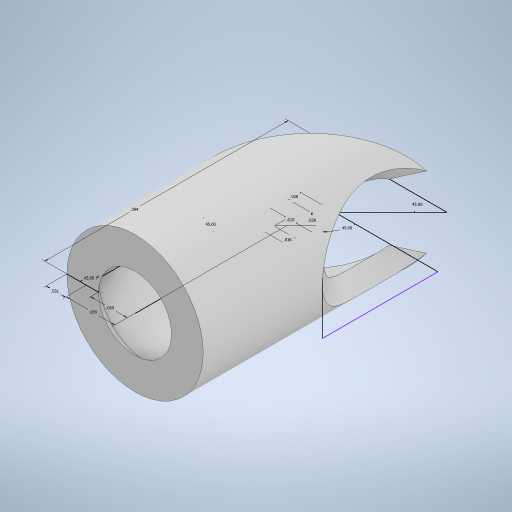
# Autodesk Inventor part: aperature
Saved by Autodesk Inventor 2024 (Build 280153000, 153)
## iProperties
Created: 2024-10-31
Part Number: aperature
Material: Generic
Document SubType Name: Modeling
Designer: Williamow
Density: 1 g/cm^3
Appearance: Default
Author: Williamow
Autodesk Inventor part; units mm, degrees
ref_plane "YZ Plane" through (0, 0, 0) normal (1, 0, 0) x (0, 1, 0)
ref_plane "XZ Plane" through (0, 0, 0) normal (0, 1, 0) x (-1, 0, 0)
ref_plane "XY Plane" through (0, 0, 0) normal (0, 0, 1) x (1, 0, 0)
sketch "Sketch1" plane through (0, 0, 0) normal (0, 1, 0) x (-1, 0, 0)
  line L0 (0, 0) -> (0, -1.3956)
  line L1 (1.5, 0) -> (2.8, 0)
  line L2 (2.8, 0) -> (2.8, -10)
  line L3 (2.8, -10) -> (2, -10)
  line L4 (2, -10) -> (2, -0.5)
  line L5 (2, -5.9601) -> (0.25, -5.9601)
  line L6 (0.25, -5.9601) -> (0.25, -5.5601)
  line L7 (0.25, -5.5601) -> (2, -3.8101)
  line L8 (2, -3.8101) -> (2, -5.9601)
  line L9 (2.8, -4.4) -> (-2.8, -10)
  line L10 (-2.8, -10) -> (2.8, -10)
  line L11 (-2.8, -10) -> (-2.0623, -10)
  line L12 (2, -0.5) -> (1.5, 0)
  line L13 (0, -7.2) -> (0, -7.7) construction
  line L14 (0, -7.7) -> (-4.7359, -7.7)
  line L15 (-4.7359, -7.7) -> (-4.7359, -2.9641)
  line L16 (-4.7359, -2.9641) -> (0, -7.7)
  point P0 (2, -3.8101)
  point P1 (0, -10)
  point P2 (2, -10)
  point P3 (2, -5.2)
  point P4 (0.9439, -6.2561)
  point P5 (1.2399, -5.9601)
  point P6 (0.2, -7)
  point P7 (2, -5.2)
  point P8 (-0.5, -7.7)
  point P9 (-0.25, -7.45)
  dimension "d1" = 10
  dimension "d4" = 2
  dimension "d10" = 45
  dimension "d19" = 0.8
  dimension "d21" = 1.5
  dimension "d23" = 45
  dimension "d24" = 45
  dimension "d25" = 0.25
  dimension "d26" = 0.4
  dimension "d27" = 0.7
  dimension "d30" = 0.5
  dimension "d31" = 45
  constraints: 34 end point, 5 horizontal, 3 parallel, 3 perpendicular, 2 midpoint, 2 point on line, 2 vertical, 1 horizontal alignment, 1 vertical alignment
  measures "d1" distance of L1.end L2.end
  measures "d4" distance between parallel lines of L0 L4
  measures "d10" angle of L10 L9
  measures "d19" distance between parallel lines of L2 L4
  measures "d21" distance of L0.start L1.start
  measures "d23" angle of L7 L8
  measures "d24" angle of L1 L12
  measures "d25" horizontal distance of L0.start L5.end
  measures "d26" distance of L5.end L6.end
  measures "d27" distance from line of L9 L5.end
  measures "d30" distance of L13.start L13.end
  measures "d31" angle of L14 L16
revolve "Revolution1" add sketch "Sketch1" angle 360 about axis through (0, 0, 0) along (0, 0, -1) contours L1 L2 L9 L4 L12 | L2 L3 L4 L9 | L4 L9 L5 L6 L7 | L4 L5 L9
extrude "Extrusion4" cut sketch "Sketch1" along normal mid plane 25.4 contours L2 L3 L4 L9 | L4 L5 L9 | L10 L9 L14 L16 L5 L4 | L16 L14 L9
revolve "Revolution3" cut sketch "Sketch1" angle 360 about axis through (0, 0, -7.7) along (1, 0, 0) contours L9 L14 L15 L16
body "Solid1"
